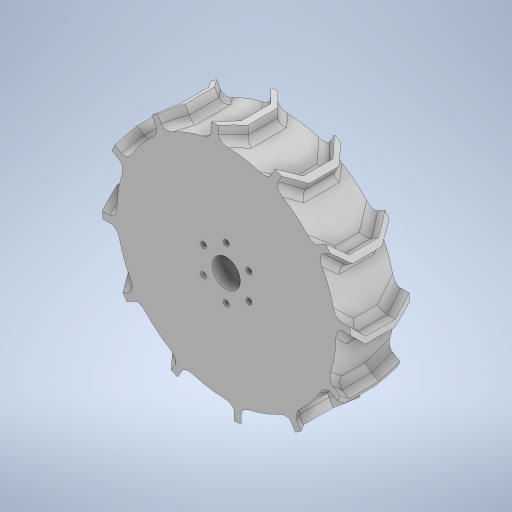
# Autodesk Inventor part: robot rubber wheels 1
Saved by Autodesk Inventor 2024 (Build 280153000, 153)
## iProperties
Created: 2024-02-14
Part Number: robot rubber wheels 1
Material: Generic
Document SubType Name: Modeling
Designer: dustp
Density: 1 g/cm^3
Appearance: Default
Author: dustp
Autodesk Inventor part; units mm, degrees
ref_plane "YZ Plane" through (0, 0, 0) normal (1, 0, 0) x (0, 1, 0)
sketch "Sketch1" plane through (0, 0, 0) normal (0, 1, 0) x (-1, 0, 0)
  circle A0 centre (0, 0) radius 46.99
  circle A1 centre (0, 0) radius 17.75
  circle A2 centre (0, 0) radius 11.25
  circle A3 centre (-8.168, 7.736) radius 1.25
  circle A4 centre (8.168, 7.736) radius 1.25
  circle A5 centre (0, -11.25) radius 1.25
  circle A6 centre (0, 0) radius 6
  dimension "d0" = 93.98
  dimension "d1" = 35.5
  dimension "d5" = 6.5
  dimension "d6" = 2.5
  dimension "d7" = 2.5
  dimension "d8" = 2.5
  dimension "d19" = 12
  constraints: 7 centre point, 3 coincident, 3 point on circle
  measures "d0" diameter of A0
  measures "d1" diameter of A1
  measures "d5" radial gap between concentric circles of A1 A2
  measures "d6" diameter of A3
  measures "d7" diameter of A4
  measures "d8" diameter of A5
  measures "d19" diameter of A6
extrude "Extrusion1" add sketch "Sketch1" along normal blind 25.4 contours A0 | A1 | A2 A5 A3 A4 | A4 A2 | A2 A4 | A5 A2 | A2 A5 | A3 A2 | A2 A3 | A6
sketch "Sketch2" plane through (0, 0, 0) normal (0, -1, 0) x (1, 0, 0)
  circle A0 centre (0, 0) radius 17.75
  circle A1 centre (0, 0) radius 11.25
  circle A2 centre (0, -11.25) radius 1.25
  dimension "d11" = 35.5
  dimension "d12" = 6.5
  dimension "d13" = 2.5
  constraints: 2 centre point, 2 coincident, 1 vertical alignment, 2 other
  measures "d11" diameter of A0
  measures "d13" diameter of A2
extrude "Extrusion2" cut sketch "Sketch1" along normal blind 25.4 contours A5 A2 | A2 A5 | A6
pattern_circular "Circular Pattern1" count 6 over 360 about axis through (0, 0, 0) along (0, 1, 0) of "Extrusion2"
ref_plane "Work Plane1" through (0, 0, 50.8) normal (0, 0, 1) x (1, 0, 0)
ref_plane "Work Plane2" through (0, 12.7, 0) normal (0, -1, 0) x (1, 0, 0)
sketch "Sketch10" plane through (0, 0, 50.8) normal (0, 0, 1) x (1, 0, 0)
  line L0 (2.9463, 19.05) -> (-0.0537, 19.05)
  line L1 (-0.0537, 19.05) -> (-0.0537, 6.35)
  line L2 (-0.0537, 6.35) -> (2.9463, 6.35)
  line L3 (2.9463, 6.35) -> (2.9463, 19.05)
  line L4 (46.99, 25.4) -> (-46.99, 25.4) projected
  line L5 (2.9463, 19.05) -> (-3.4037, 25.4)
  line L6 (2.9463, 19.05) -> (11.9265, 19.05) construction
  line L7 (-0.0537, 19.05) -> (-6.4037, 25.4)
  line L8 (-0.0537, 19.05) -> (8.9265, 19.05) construction
  line L9 (-6.4037, 25.4) -> (-3.4037, 25.4)
  line L10 (-0.0537, 6.35) -> (-6.4037, 0)
  line L11 (2.9463, 6.35) -> (-3.4037, 0)
  line L12 (46.99, 0) -> (-46.99, 0) projected
  line L13 (2.9463, 6.35) -> (11.9265, 6.35) construction
  line L14 (-3.4037, 0) -> (-6.4037, 0)
  dimension "d81" = 3
  dimension "d82" = 12.7
  dimension "d83" = 6.35
  dimension "d84" = 135
  dimension "d85" = 135
  dimension "d86" = 135
  constraints: 26 end point, 5 horizontal, 3 equal length, 3 point on line, 2 parallel, 2 perpendicular
  measures "d81" distance of L0.start L0.end
  measures "d82" distance of L2.end L0.start
  measures "d83" distance between parallel lines of L4 L0
  measures "d84" angle of L6 L5
  measures "d85" angle of L8 L7
  measures "d86" angle of L11 L13
extrude "Extrusion7" add sketch "Sketch10" along normal blind 3 and the other way blind 5
fillet "Fillet3" radius 3 6 edges at (-0.2292, 3.1745, 46.9894) (2.9463, 12.7, 46.8975) (-0.2292, 22.2255, 46.9894) (-3.2362, 22.2324, 46.8784) (-0.0537, 12.7, 46.99) (-3.2362, 3.1676, 46.8784)
pattern_circular "Circular Pattern4" count 12 over 360 about axis through (0, 0, 0) along (0, 1, 0) of "Extrusion7", "Fillet3"
sketch "Sketch11" plane through (0, 0, 0) normal (0, -1, 0) x (1, 0, 0)
  arc A0 (-6, 0) -> (-3, -5.1962) centre (0, 0) ccw projected
  circle A1 centre (0, 0) radius 53.34
  dimension "d99" = 106.68
  constraints: 1 centre point, 1 coincident
  measures "d99" diameter of A1
extrude "Extrusion8" cut sketch "Sketch11" against normal blind 25.4 keep common part
sketch "Sketch12" plane through (0, 0, 0) normal (0, -1, 0) x (1, 0, 0)
  point P0 (0, 0)
body "Solid1"
